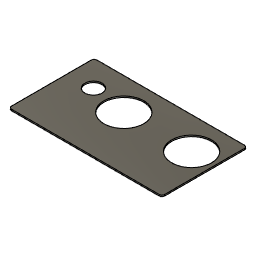
Top_v3 (Autodesk Fusion 360 design; units mm, degrees)
Autodesk Fusion 360 part; units mm, degrees
sketch "Esquisse1" plane through (0, 0, 0) normal (0, 0, 1) x (1, 0, 0)
  line L0 (74.9967, -34.0812) -> (-36.2033, -34.0812)
  circle A0 centre (59.0467, 6.2188) radius 15
  line L1 (76.9967, 28.1188) -> (76.9967, -32.0812)
  line L2 (-38.2033, -32.0812) -> (-38.2033, 28.1188)
  line L3 (74.8967, -31.9812) -> (-36.1033, -31.9812)
  line L4 (-36.2033, 30.1188) -> (74.9967, 30.1188)
  line L5 (-36.1033, 28.0188) -> (74.8967, 28.0188)
  line L6 (-36.1033, -31.9812) -> (-36.1033, 28.0188)
  circle A1 centre (8.0467, 6.2188) radius 15
  line L7 (74.8967, 28.0188) -> (74.8967, -31.9812)
  arc A2 (74.9967, -34.0812) -> (76.9967, -32.0812) centre (74.9967, -32.0812) ccw
  arc A3 (76.9967, 28.1188) -> (74.9967, 30.1188) centre (74.9967, 28.1188) ccw
  arc A4 (-36.2033, 30.1188) -> (-38.2033, 28.1188) centre (-36.2033, 28.1188) ccw
  arc A5 (-38.2033, -32.0812) -> (-36.2033, -34.0812) centre (-36.2033, -32.0812) ccw
  circle A6 centre (-19.1033, 10.5188) radius 6.5
  point P0 (-37.2797, 0.2421)
  dimension "d25" = 115.2
  dimension "d26" = 64.2
  dimension "d38" = 30
  dimension "d41" = 46.25
  dimension "d42" = 111
  dimension "d43" = 60
  dimension "d44" = 2.1
  dimension "d45" = 2.1
  dimension "d47" = 30
  dimension "d48" = 51
  dimension "d21" = 2
  dimension "d22" = 2
  dimension "d23" = 2
  dimension "d24" = 2
  dimension "d28" = 13
  dimension "d29" = 42.5
  dimension "d30" = 17
  dimension "d34" = 38.2
  dimension "d35" = 38.2
  constraint horizontal L4
  constraint vertical L1
  constraint horizontal L0
  constraint vertical L2
  constraint horizontal L5
  constraint vertical L7
  constraint horizontal L3
  constraint vertical L6
  constraint tangent L0 A2
  constraint tangent L1 A2
  constraint tangent L4 A3
  constraint tangent L1 A3
  constraint tangent L2 A4
  constraint tangent L4 A4
  constraint tangent L2 A5
  constraint tangent L0 A5
  measures "d25" distance of L1 L2
  measures "d26" distance of L0 L4
  measures "d38" diameter of A1
  measures "d41" distance of A1.centre L2
  measures "d42" distance of L5.end L5.start
  measures "d43" distance of L3.end L5.start
  measures "d44" distance of L2 L6
  measures "d45" distance of L4 L5
  measures "d47" diameter of A0
  measures "d48" horizontal distance of A0.centre A1.centre
  measures "d21" radius of A2
  measures "d22" radius of A3
  measures "d23" radius of A4
  measures "d24" radius of A5
  measures "d28" diameter of A6
  measures "d29" distance of L3 A6.centre
  measures "d30" distance of L6 A6.centre
  measures "d34" distance of A0.centre L3
  measures "d35" distance of A1.centre L3
extrude "Extrusion1" add sketch "Esquisse1" along normal blind 1 contours L0 L1 L2 L4 A2 A3 A4 A5 | L3 L5 L6 L7
